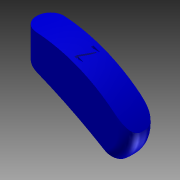
# Autodesk Inventor part: Z Button
Saved by Autodesk Inventor 2012 SP1 (Build 160190100, 190)
## iProperties
Created: 2011-12-13
Part Number: Z Button
Material: Default
Document SubType Name: Modeling
Designer: 133098
Density: 1 g/cm^3
Author: 133098
Autodesk Inventor part; units mm, degrees
ref_plane "YZ Plane" through (0, 0, 0) normal (1, 0, 0) x (0, 1, 0)
ref_plane "XZ Plane" through (0, 0, 0) normal (0, 1, 0) x (-1, 0, 0)
ref_plane "XY Plane" through (0, 0, 0) normal (0, 0, 1) x (1, 0, 0)
sketch "Sketch1" plane through (0, 0, 0) normal (0, 0, 1) x (1, 0, 0)
  line L0 (21.0058, 10.4287) -> (21.0058, 17.0196)
  arc A0 (42.0116, 0.0645) -> (21.0058, 10.4287) centre (-15.493, -90.014) ccw
  arc A1 (45.1866, 6.5935) -> (21.0058, 17.0196) centre (22.2535, -13.3404) ccw
  arc A2 (42.0116, 0.0645) -> (45.1866, 6.5935) centre (36.8861, 6.5935) ccw
  point P0 (42.0116, 0)
  constraints: 6 point on circle, 3 centre point, 2 end point
extrude "Extrusion1" add sketch "Sketch1" along normal blind 6.35
fillet "Fillet1" radius 3.175 2 edges at (21.0058, 13.7242, 6.35) (21.0058, 13.7242, 0)
fillet "Fillet2" radius 2.6426 2 edges at (44.3508, 2.9634, 6.35) (44.3508, 2.9634, 0)
sketch "Sketch2" plane through (0, 0, 0) normal (0, 1, 0) x (-1, 0, 0)
  line L0 (-33.3094, 5.3628) -> (-27.2705, 5.3628) construction
  line L1 (-27.2705, 5.3628) -> (-27.2705, 1.5536) construction
  line L2 (-27.2705, 1.5536) -> (-33.3094, 1.5536) construction
  line L3 (-33.3094, 1.5536) -> (-33.3094, 5.3628) construction
  line L4 (-31.7138, 1.0448) -> (-33.2219, 1.0448)
  line L5 (-33.2219, 1.0448) -> (-33.2219, 1.5802)
  line L6 (-33.2219, 1.5802) -> (-32.0637, 4.8519)
  line L7 (-32.0637, 4.8519) -> (-33.1694, 4.8519)
  line L8 (-33.1694, 4.8519) -> (-33.1694, 5.3628)
  line L9 (-33.1694, 5.3628) -> (-31.7418, 5.3628)
  line L10 (-31.7418, 5.3628) -> (-31.7418, 4.8449)
  line L11 (-31.7418, 4.8449) -> (-32.9105, 1.5557)
  line L12 (-32.9105, 1.5557) -> (-31.7138, 1.5557)
  line L13 (-31.7138, 1.5557) -> (-31.7138, 1.0448)
  point P0 (0, 0)
  constraints: 2 other
extrude "Extrusion2" add sketch "Sketch2" along normal blind 16.51
sketch "Sketch3" plane through (0, 0, 0) normal (0, -1, 0) x (1, 0, 0)
  line L0 (31.7138, 1.0448) -> (33.2219, 1.0448) projected
  line L1 (33.2219, 1.0448) -> (33.2219, 1.5802) projected
  line L2 (33.2219, 1.5802) -> (32.0637, 4.8519) projected
  line L3 (32.0637, 4.8519) -> (33.1694, 4.8519) projected
  line L4 (33.1694, 4.8519) -> (33.1694, 5.3628) projected
  line L5 (33.1694, 5.3628) -> (31.7418, 5.3628) projected
  line L6 (31.7418, 5.3628) -> (31.7418, 4.8449) projected
  line L7 (31.7418, 4.8449) -> (32.9105, 1.5557) projected
  line L8 (32.9105, 1.5557) -> (31.7138, 1.5557) projected
  line L9 (31.7138, 1.5557) -> (31.7138, 1.0448) projected
  point P0 (0, 0)
extrude "Extrusion3" cut sketch "Sketch3" against normal up to surface round surface about axis through (-15.493, -90.014, 0) along (0, 0, 1) radius 106.8686 far side no
sketch "Sketch4" plane through (0, 16.51, 0) normal (0, 1, 0) x (1, 0, 0)
  line L0 (33.2219, -1.0448) -> (33.2219, -1.5802) projected
  line L1 (31.7138, -1.0448) -> (33.2219, -1.0448) projected
  line L2 (31.7138, -1.5557) -> (31.7138, -1.0448) projected
  line L3 (32.9105, -1.5557) -> (31.7138, -1.5557) projected
  line L4 (31.7418, -4.8449) -> (32.9105, -1.5557) projected
  line L5 (31.7418, -5.3628) -> (31.7418, -4.8449) projected
  line L6 (33.1694, -5.3628) -> (31.7418, -5.3628) projected
  line L7 (33.1694, -4.8519) -> (33.1694, -5.3628) projected
  line L8 (32.0637, -4.8519) -> (33.1694, -4.8519) projected
  line L9 (33.2219, -1.5802) -> (32.0637, -4.8519) projected
  point P0 (0, 0)
extrude "Extrusion4" cut sketch "Sketch4" against normal blind 1.5875
sketch "Sketch5" plane through (31.7138, 14.9225, 1.0448) normal (0, 0, 1) x (1, 0, 0)
  line L0 (0, 0.6125) -> (0, 0) projected
  line L1 (1.5082, 0) -> (0, 0) projected
  line L2 (1.5082, 0) -> (0, 0.3062)
  line L3 (0, 0.3062) -> (0, 0)
  point P0 (-31.7138, -14.9225)
  constraints: 4 end point, 1 midpoint, 1 perpendicular
extrude "Extrusion5" [suppressed]
sketch "Sketch6" plane through (32.9105, 14.9225, 1.5557) normal (0, 0, 1) x (1, 0, 0)
  line L0 (0, 0.0632) -> (0, 0) projected
  line L1 (0.3114, 0) -> (0, 0) projected
  line L2 (0, 0.0632) -> (0.3114, 0) projected
  point P0 (-32.9105, -14.9225)
extrude "Extrusion6" [suppressed]
body "Solid1"
